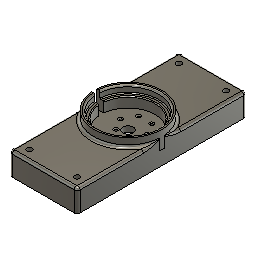
StaticBase v19 (Autodesk Fusion 360 design; units mm, degrees)
Autodesk Fusion 360 part; units mm, degrees
note: some values were not read from the file. Set by a fixed rule: which sketch regions a step uses.
sketch "Sketch1" plane through (0, 0, 0) normal (0, 1, 0) x (-1, 0, 0)
  circle A0 centre (7.75, 53.037581) radius 1.5
  circle A1 centre (7.75, 26.190794) radius 1.5
  circle A2 centre (-15.5, 39.614187) radius 1.5
  circle A3 centre (-7.75, 26.190794) radius 1.5
  circle A4 centre (15.5, 39.614187) radius 1.5
  circle A5 centre (-7.75, 53.037581) radius 1.5
  circle A6 centre (0, 46.614187) radius 6
  circle A7 centre (-15.5, 39.614187) radius 1.6
  circle A8 centre (-7.75, 53.037581) radius 1.6
  circle A9 centre (7.75, 53.037581) radius 1.6
  circle A10 centre (15.5, 39.614187) radius 1.6
  circle A11 centre (7.75, 26.190794) radius 1.6
  circle A12 centre (-7.75, 26.190794) radius 1.6
  circle A13 centre (0, 46.614187) radius 6.15
  line L0 (40, 39.614187) -> (40, 146.614187)
  line L1 (-40, 39.614187) -> (-40, 146.614187)
  line L2 (-40, 39.614187) -> (-40, -53.385813)
  line L3 (-40, -53.385813) -> (40, -53.385813)
  line L4 (40, -53.385813) -> (40, 39.614187)
  line L5 (40, 146.614187) -> (-40, 146.614187)
  line L6 (40, -13.385813) -> (-40, -13.385813)
  line L7 (40, 106.614187) -> (-40, 106.614187)
  line L8 (0, 150) -> (0, -80) construction
  line L9 (46.540026, 46.614187) -> (-48.931314, 46.614187) construction
  circle A14 centre (0, 39.614187) radius 15.5
  line L10 (35, -13.385813) -> (35, 106.614187)
  line L11 (-35, -13.385813) -> (-35, 106.614187)
  dimension "d24" = 40
  dimension "d25" = 40
  dimension "d5" = 100
  dimension "d6" = 100
  dimension "d11" = 12.3
  dimension "d12" = 3.2
  dimension "d13" = 3.2
  dimension "d14" = 3.2
  dimension "d15" = 3.2
  dimension "d16" = 3.2
  dimension "d17" = 3.2
  dimension "d18" = 15.5
  dimension "d19" = 7
  dimension "d28" = 31
  dimension "d29" = 7
  dimension "d31" = 40
  dimension "d32" = 40
  dimension "d35" = 5
  dimension "d36" = 5
  constraint concentric A5 A8
  constraint concentric A0 A9
  constraint concentric A1 A11
  constraint concentric A3 A12
  constraint concentric A6 A13
  constraint vertical L0
  constraint vertical L1
  constraint perpendicular L0 L3
  constraint perpendicular L3 L4
  constraint perpendicular L0 L5
  constraint perpendicular L2 L6
  constraint perpendicular L1 L7
  constraint perpendicular L5 L8
  constraint perpendicular L1 L9
  constraint symmetric A7 A10 L8
  constraint perpendicular L7 L10
  constraint perpendicular L7 L11
  measures "d24" distance of L3 L6
  measures "d25" distance of L5 L7
  measures "d5" distance of L3 L9
  measures "d6" distance of L5 L9
  measures "d11" diameter of A13
  measures "d12" diameter of A9
  measures "d13" diameter of A10
  measures "d14" diameter of A11
  measures "d15" diameter of A12
  measures "d16" diameter of A7
  measures "d17" diameter of A8
  measures "d28" diameter of A14
  measures "d31" distance of L4 L8
  measures "d32" distance of L2 L8
  measures "d35" distance of L0 L10
  measures "d36" distance of L1 L11
extrude "Extrude7" add sketch "Sketch1" along normal blind 6.5 contours A7 A8 A9 A10 A11 A12 A14 | L0 L4 L6 L7 L10 | L0 L1 L5 L7 | L2 L3 L4 L6 | L6 L7 L10 L11 | L1 L2 L6 L7 L11 picked at (7.996831, 33.64073) picked at (36.666667, 44.280854) picked at (-11.666667, 133.280854) picked at (-11.666667, -40.052479) picked at (0, 89.447521) picked at (-36.666667, 44.280854)
extrude "Extrude8" add sketch "Sketch1" against normal blind 10 contours L0 L4 L6 L7 L10 | L0 L1 L5 L7 | L2 L3 L4 L6 | L1 L2 L6 L7 L11 picked at (36.666667, 44.280854) picked at (-11.666667, 133.280854) picked at (-11.666667, -40.052479) picked at (-36.666667, 44.280854)
sketch "Sketch3" plane through (0, 6.5, 0) normal (0, 1, 0) x (-1, 0, 0)
  circle A0 centre (7.75, 26.190794) radius 1.6
  circle A1 centre (15.5, 39.614187) radius 1.6
  circle A2 centre (0, 46.614187) radius 6.15
  circle A3 centre (7.75, 53.037581) radius 1.6
  circle A4 centre (-7.75, 26.190794) radius 1.6
  circle A5 centre (-15.5, 39.614187) radius 1.6
  circle A6 centre (-7.75, 53.037581) radius 1.6
  line L0 (-40, 146.614187) -> (-40, -53.385813)
  line L1 (-40, -53.385813) -> (40, -53.385813)
  line L2 (40, -53.385813) -> (40, 146.614187)
  line L3 (40, 146.614187) -> (-40, 146.614187)
  circle A7 centre (0, 46.614187) radius 31.75
  circle A8 centre (0, 46.614187) radius 40
  line L4 (31.75, 46.614187) -> (40, 46.614187) construction
  line L5 (31.60795, 49.614187) -> (39.887341, 49.614187)
  line L6 (31.60795, 43.614187) -> (39.887341, 43.614187)
  dimension "d39" = 63.5
  dimension "d41" = 3
  constraint concentric A2 A7
  constraint concentric A7 A8
  constraint tangent L2 A8
  constraint perpendicular L2 L4
  constraint perpendicular L2 L5
  measures "d39" diameter of A7
  measures "d41" distance of L4 L5
extrude "Extrude9" add sketch "Sketch3" along normal blind 12 contours A7 A8 L5 L6 picked at (-37.078885, 43.888312)
sketch "Sketch4" plane through (0, 18.5, 0) normal (0, 1, 0) x (-1, 0, 0)
  line L0 (31.60795, 49.614187) -> (39.887341, 49.614187)
  arc A0 (39.887341, 49.614187) -> (39.887341, 43.614187) centre (0, 46.614187) ccw
  line L1 (39.887341, 43.614187) -> (31.60795, 43.614187)
  arc A1 (31.60795, 49.614187) -> (31.60795, 43.614187) centre (0, 46.614187) ccw
  circle A2 centre (0, 46.614187) radius 36.15
  dimension "d44" = 72.3
  constraint concentric A0 A2
  measures "d44" diameter of A2
extrude "Extrude10" add sketch "Sketch4" along normal blind 8.5 contours L0 A0 L1 A2 picked at (38.30249, 51.58448)
fillet "Fillet6" radius 1 6 edges at (16.991724, 6.5, 40.192772) (9.241724, 6.5, 53.616166) (9.241724, 6.5, 26.769378) (-6.258276, 6.5, 26.769378) (-14.008276, 6.5, 40.192772) (-6.258276, 6.5, 53.616166)
fillet "Fillet7" radius 1 2 edges at (31.75, 18.5, 46.614187) (36.15, 18.5, 46.614187)
fillet "Fillet8" radius 2 1 edges at (36.15, 27, 46.614187)
sketch "Sketch5" plane through (0, 6.5, 0) normal (0, 1, 0) x (-1, 0, 0)
  line L0 (40, -53.385813) -> (40, 146.614187)
  line L1 (40, 146.614187) -> (-40, 146.614187)
  line L2 (-40, 146.614187) -> (-40, 46.614187)
  circle A0 centre (28, 134.614187) radius 3.1
  line L3 (0, 160.139832) -> (0, -64.91971) construction
  line L4 (38.031862, 43.614187) -> (36.025304, 43.614187)
  line L5 (36.025304, 49.614187) -> (38.031862, 49.614187)
  line L6 (42.850808, 46.614187) -> (-49.000001, 46.614187) construction
  line L7 (35.021743, 43.614187) -> (32.612306, 43.614187)
  line L8 (32.612306, 49.614187) -> (35.021743, 49.614187)
  circle A1 centre (-7.75, 53.037581) radius 1.6
  circle A2 centre (7.75, 53.037581) radius 1.6
  circle A3 centre (-28, 134.614187) radius 3.1
  circle A4 centre (-28, -41.385813) radius 3.1
  circle A5 centre (28, -41.385813) radius 3.1
  circle A6 centre (15.5, 39.614187) radius 2.6
  circle A7 centre (-7.75, 26.190794) radius 2.6
  circle A8 centre (-15.5, 39.614187) radius 2.6
  arc A9 (39.887341, 49.614187) -> (-40, 46.614187) centre (0, 46.614187) ccw
  line L9 (39.887341, 49.614187) -> (31.60795, 49.614187)
  arc A10 (31.60795, 49.614187) -> (31.60795, 43.614187) centre (0, 46.614187) ccw
  line L10 (31.60795, 43.614187) -> (39.887341, 43.614187)
  arc A11 (-40, 46.614187) -> (39.887341, 43.614187) centre (0, 46.614187) ccw
  line L11 (-40, 46.614187) -> (-40, -53.385813)
  line L12 (-40, -53.385813) -> (40, -53.385813)
  circle A12 centre (0, 46.614187) radius 6.15
  circle A13 centre (-7.75, 53.037581) radius 2.6
  circle A14 centre (7.75, 26.190794) radius 2.6
  circle A15 centre (7.75, 53.037581) radius 2.6
  circle A16 centre (0, 46.614187) radius 40
  line L13 (39.887341, 43.614187) -> (40, 43.614187)
  line L14 (39.887341, 49.614187) -> (40, 49.614187)
  line L15 (-39.887341, 43.614187) -> (-40, 43.614187)
  line L16 (-39.887341, 49.614187) -> (-40, 49.614187)
  dimension "d55" = 6.2
  dimension "d56" = 12
  dimension "d57" = 12
  dimension "d60" = 3
  dimension "d62" = 6
  dimension "d63" = 3.2
  dimension "d64" = 3.2
  dimension "d65" = 15.5
  dimension "d66" = 7.75
  constraint perpendicular L1 L3
  constraint horizontal L6
  constraint symmetric A0 L3 A3
  constraint symmetric A0 L6 A5
  constraint symmetric L6 A3 A4
  constraint concentric A9 A16
  constraint perpendicular L0 L13
  measures "d55" diameter of A0
  measures "d60" distance of L6 L7
  measures "d62" distance of L7 L8
  measures "d63" diameter of A1
  measures "d64" diameter of A2
extrude "Extrude11" cut sketch "Sketch5" against normal blind 16.5 contours A0 | A3 | A4 | A5 picked at (27.483333, 132.822601) picked at (-28.516667, 132.822601) picked at (-29.390878, -41.834159) picked at (26.609122, -41.834159)
extrude "Extrude12" add sketch "Sketch5" along normal blind 10 contours L0 A11 L11 L12 A16 L13 L15 | L0 L1 L2 A9 A16 L14 L16 picked at (0, -24.221618) picked at (0, 117.449993)
fillet "Fillet9" radius 3.5 4 edges at (40, 3.25, 146.614187) (-40, 3.25, 146.614187) (40, 3.25, -53.385813) (-40, 3.25, -53.385813)
fillet "Fillet10" radius 3 12 edges at (0, 16.5, 6.614187) (0, 16.5, 86.614187) (-40, 16.5, 96.364187) (-38.974874, 16.5, 145.589061) (0, 16.5, 146.614187) (38.974874, 16.5, 145.589061) (40, 16.5, 96.364187) (40, 16.5, -3.135813) (38.974874, 16.5, -52.360686) (0, 16.5, -53.385813) (-38.974874, 16.5, -52.360686) (-40, 16.5, -3.135813)
equation "d25 = d24"
equation "d6 = d5"
equation "d13 = d12"
equation "d14 = d12"
equation "d15 = d12"
equation "d16 = d12"
equation "d17 = d12"
equation "d32 = d31"
equation "d36 = d35"
equation "d39 = ( ( 72 - 55 ) / 2 ) * 1 mm + 55 mm"
equation "d56 = ( d55 - 0.2 mm ) * 2"
equation "d57 = d56"
equation "d66 = d65 / 2"
